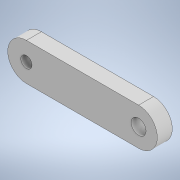
# Autodesk Inventor part: horn slider pen
Saved by Autodesk Inventor 2020 (Build 240168000, 168)
## iProperties
Created: 2026-07-08
Part Number: horn slider pen
Material: Generic
Document SubType Name: Modeling
Designer: drago
Density: 1 g/cm^3
Appearance: Default
Author: drago
Autodesk Inventor part; units mm, degrees
ref_plane "YZ Plane" through (0, 0, 0) normal (1, 0, 0) x (0, 1, 0)
ref_plane "XZ Plane" through (0, 0, 0) normal (0, 1, 0) x (-1, 0, 0)
ref_plane "XY Plane" through (0, 0, 0) normal (0, 0, 1) x (1, 0, 0)
sketch "Sketch1" plane through (0, 0, 0) normal (0, 0, 1) x (1, 0, 0)
  line L0 (0, 0) -> (15, 0) construction
  line L1 (0, -2.5) -> (15, -2.5)
  line L2 (15, 2.5) -> (0, 2.5)
  arc A0 (0, 2.5) -> (0, -2.5) centre (0, 0) ccw
  arc A1 (15, -2.5) -> (15, 2.5) centre (15, 0) ccw
  circle A2 centre (15, 0) radius 1
  circle A3 centre (0, 0) radius 1
  point P0 (7.5, 0)
  dimension "d0" = 15
  dimension "d1" = 5
  dimension "d2" = 2
  dimension "d3" = 2
  constraints: 8 end point, 4 centre point, 4 point on circle, 4 tangent, 2 coincident, 1 horizontal, 1 midpoint, 1 parallel
  measures "d0" distance of L0.start L0.end
  measures "d1" diameter of A1
  measures "d2" diameter of A2
  measures "d3" diameter of A3
extrude "Extrusion1" add sketch "Sketch1" along normal blind 2
sketch "Sketch2" plane through (0, 0, 2) normal (0, 0, 1) x (1, 0, 0)
  circle A0 centre (0, 0) radius 0.75
  circle A1 centre (0, 0) radius 1
  dimension "d6" = 1.5
  constraints: 2 centre point, 2 coincident
  measures "d6" diameter of A0
extrude "Extrusion2" add sketch "Sketch2" against normal blind 2
body "Solid1"
